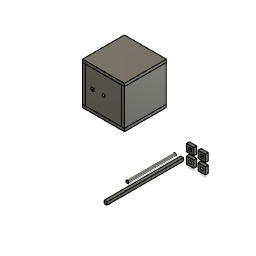
05-joint-revolute-slider-practice (Autodesk Fusion 360 design; units mm, degrees)
Autodesk Fusion 360 part; units mm, degrees
sketch "スケッチ1" plane through (0, 0, 0) normal (0, 0, 1) x (1, 0, 0)
  line L0 (0, 0) -> (25, 0)
  line L1 (25, 0) -> (25, 25)
  line L2 (25, 25) -> (0, 25)
  line L3 (0, 25) -> (0, 0)
  line L4 (30, 25) -> (55, 25)
  line L5 (55, 25) -> (55, 0)
  line L6 (55, 0) -> (30, 0)
  line L7 (30, 0) -> (30, 25)
  line L8 (0, 59) -> (29, 59)
  line L9 (29, 59) -> (29, 30)
  line L10 (29, 30) -> (0, 30)
  line L11 (0, 30) -> (0, 59)
  line L12 (30, 30) -> (59, 30)
  line L13 (59, 30) -> (59, 59)
  line L14 (59, 59) -> (30, 59)
  line L15 (30, 59) -> (30, 30)
  line L16 (0, 65) -> (29, 65)
  line L17 (29, 65) -> (29, 90)
  line L18 (29, 90) -> (0, 90)
  line L19 (0, 90) -> (0, 65)
  line L20 (30, 90) -> (59, 90)
  line L21 (59, 90) -> (59, 65)
  line L22 (59, 65) -> (30, 65)
  line L23 (30, 65) -> (30, 90)
  circle A0 centre (12.5, 12.5) radius 1
  circle A1 centre (42.5, 12.5) radius 1
  line L24 (4, 13.5) -> (6, 13.5)
  line L25 (6, 13.5) -> (6, 11.5)
  line L26 (6, 11.5) -> (4, 11.5)
  line L27 (4, 11.5) -> (4, 13.5)
  line L28 (49, 13.5) -> (51, 13.5)
  line L29 (51, 13.5) -> (51, 11.5)
  line L30 (51, 11.5) -> (49, 11.5)
  line L31 (49, 11.5) -> (49, 13.5)
  circle A2 centre (60, 0) radius 1
  line L32 (64, 1) -> (66, 1)
  line L33 (66, 1) -> (66, -1)
  line L34 (66, -1) -> (64, -1)
  line L35 (64, -1) -> (64, 1)
  line L36 (70, 5) -> (75, 5)
  line L37 (75, 5) -> (75, 0)
  line L38 (75, 0) -> (70, 0)
  line L39 (70, 0) -> (70, 5)
  circle A3 centre (72.5, 2.5) radius 1
  line L40 (70, 12.5) -> (75, 12.5)
  line L41 (75, 12.5) -> (75, 7.5)
  line L42 (75, 7.5) -> (70, 7.5)
  line L43 (70, 7.5) -> (70, 12.5)
  line L44 (73.5, 11) -> (71.5, 11)
  line L45 (71.5, 11) -> (71.5, 9)
  line L46 (71.5, 9) -> (73.5, 9)
  line L47 (73.5, 9) -> (73.5, 11)
  line L48 (73.5, 11) -> (71.5, 9) construction
  line L49 (71.5, 11) -> (73.5, 9) construction
  point P0 (72.5, 10)
  dimension "d13" = 2
  constraint horizontal L0
  constraint vertical L1
  constraint horizontal L2
  constraint vertical L3
  constraint coincident L0.start L3.end
  constraint horizontal L4
  constraint vertical L5
  constraint horizontal L6
  constraint vertical L7
  constraint horizontal L8
  constraint vertical L9
  constraint horizontal L10
  constraint vertical L11
  constraint horizontal L12
  constraint vertical L13
  constraint horizontal L14
  constraint vertical L15
  constraint horizontal L16
  constraint vertical L17
  constraint horizontal L18
  constraint vertical L19
  constraint horizontal L20
  constraint vertical L21
  constraint horizontal L22
  constraint vertical L23
  constraint horizontal L24
  constraint vertical L25
  constraint horizontal L26
  constraint vertical L27
  constraint horizontal L28
  constraint vertical L29
  constraint horizontal L30
  constraint vertical L31
  constraint horizontal L32
  constraint vertical L33
  constraint horizontal L34
  constraint vertical L35
  constraint horizontal L36
  constraint vertical L37
  constraint horizontal L38
  constraint vertical L39
  constraint horizontal L40
  constraint vertical L41
  constraint horizontal L42
  constraint vertical L43
  constraint horizontal L44
  constraint perpendicular L44 L45
  constraint parallel L44 L46
  constraint parallel L45 L47
  constraint coincident L48 P0
  constraint coincident L49 P0
  measures "d13" diameter of A0
extrude "押し出し1" add sketch "スケッチ1" along normal blind 2 contours L0 L1 L2 L3 makes body 1 in component "前"
extrude "押し出し1'" add sketch "スケッチ1" along normal blind 2 separate body contours L4 L5 L6 L7 makes body 2 in component "後"
extrude "押し出し1''" add sketch "スケッチ1" along normal blind 2 separate body contours L8 L9 L10 L11 makes body 3 in component "上"
extrude "押し出し1'''" add sketch "スケッチ1" along normal blind 2 separate body contours L12 L13 L14 L15 makes body 4 in component "下"
extrude "押し出し1''''" add sketch "スケッチ1" along normal blind 2 separate body contours L16 L17 L18 L19 makes body 5 in component "左"
extrude "押し出し1'''''" add sketch "スケッチ1" along normal blind 2 separate body contours L20 L21 L22 L23 makes body 6 in component "右"
extrude "押し出し1''''''" add sketch "スケッチ1" along normal blind 53 separate body contours L32 L33 L34 L35 makes body 7 in component "スライド軸"
extrude "押し出し1'''''''" add sketch "スケッチ1" along normal blind 33 separate body contours A2 makes body 8 in component "回転軸"
extrude "押し出し1''''''''" add sketch "スケッチ1" along normal blind 2 separate body contours L36 L37 L38 L39 makes body 9 in component "回転軸止め輪"
extrude "押し出し1'''''''''" add sketch "スケッチ1" along normal blind 2 separate body contours L40 L41 L42 L43 makes body 10 in component "スライド軸止め輪"
component "前" placed x (1, 0, 0) y (0, 1, 0) z (0, 0, 1) at (0, 0, 0)
component "後" placed x (-1, 0, 0) y (0, 1, 0) z (0, 0, -1) at (55, 0, -25)
component "上" placed x (1, 0, 0) y (0, 0, -1) z (0, 1, 0) at (-2, 25, 32)
component "下" placed x (1, 0, 0) y (0, 0, -1) z (0, 1, 0) at (-32, -2, 32)
component "左" placed x (0, 0, -1) y (0, 1, 0) z (1, 0, 0) at (-2, -65, 2)
component "右" placed x (0, 0, 1) y (0, 1, 0) z (-1, 0, 0) at (27, -65, -57)
component "スライド軸" placed x (1, 0, 0) y (0, 1, 0) z (0, 0, 1) at (0, 0, 0)
component "回転軸" placed x (1, 0, 0) y (0, 1, 0) z (0, 0, 1) at (0, 0, 0)
component "回転軸止め輪" placed x (1, 0, 0) y (0, 1, 0) z (0, 0, 1) at (0, 0, 0)
component "回転軸止め輪" placed x (1, 0, 0) y (0, 1, 0) z (0, 0, 1) at (8, 0, 0)
component "スライド軸止め輪" placed x (1, 0, 0) y (0, 1, 0) z (0, 0, 1) at (0, 0, 0)
component "スライド軸止め輪" placed x (1, 0, 0) y (0, 1, 0) z (0, 0, 1) at (8, 0, 0)
